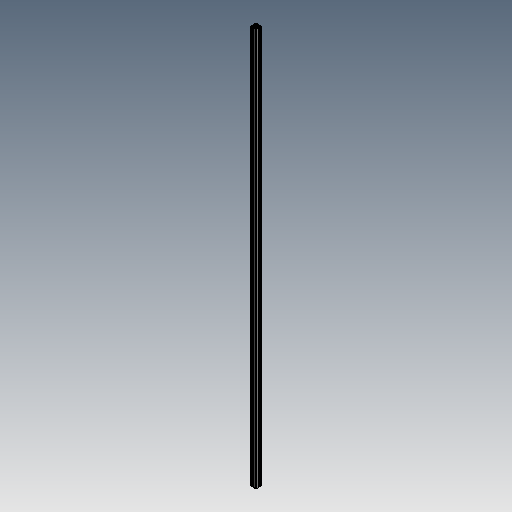
# Autodesk Inventor part: EFS6-3030-2043
Saved by Autodesk Inventor 2020 (Build 240168000, 168)
## iProperties
Part Number: EFS6-3030-2043
Material: 一般
Catalog Web Link: www.cadenas.de
Description: NEFS6-3030, NEFSB6-3030, EFS6-3030, EFSB6-3030, HFS6-3030, HFSB6-3030, CAF6-3030, HFSY6-3030, NFSL6-3030,  HFSL6-3030, HFSLB6-3030, GFS6-3030-HFS6 Series Aluminum Extrusions 30 Square -1 Slot-
Vendor: MISUMI
Document SubType Name: Modeling
Designer: partserver
Manufacturer: MISUMI
Mass: 604.165 g
Surface Area: 6959.94 cm^2
Volume: 604.165 cm^3
Density: 1 g/cm^3
Appearance: PSOLRGB-175-175-175
Category: PARTsolutions
Company: MISUMI
PSOL_IDENT_0: {$CADENAS_DATA\23d-libs\misumi\metric\38_al_extrusions_blackets\6\hfs6_3030.prj},722 {VTYP=3D},{NB=E
PSOL_IDENT_1: FS6-3030-2043},{LINA=EFS6-3030-2043},{NN=NEFS6-3030, NEFSB6-3030, EFS6-3030, EFSB6-3030, HFS6-3030,
PSOL_IDENT_2: HFSB6-3030, CAF6-3030, HFSY6-3030, NFSL6-3030,  HFSL6-3030, HFSLB6-3030, GFS6-3030},{DATE=30.06.2021
PSOL_IDENT_3: 13:36:38},{GEOMDATE=28.10.2014 00:00:00},{VERSION=},{LINEID=150},{WBVAR=L,ALT1,ALT2,ALT3,ALT4,ALT5,
PSOL_IDENT_4: CP5,DL5,DR5,ALT6,ALT9,ALT10,ALT11,DD6SE,DD6,HP6,NHL6,DL6,NHR6,DR6,ALT7,ALT8,NH9,AH,BH,CH,DH,EH,NH10,
PSOL_IDENT_5: AV,BV,CV,DV,EV,NH11,AP,BP,CP,DP,EP,ALT12,ALT13,Z,NH12,XA,XB,XC,XD,XE,NH13,YA,YB,YC,YD,YE,ALT14,HP14,
PSOL_IDENT_6: DL14,DR14,ALT15,HP15,DL15,DR15,ALT16,HP16,DL16,DR16,ALT17,HQ17,JLP,ALT19,ALT20},{WBNUMERIC=L,DD6,NH9
PSOL_IDENT_7: ,AH,BH,CH,DH,EH,NH10,AV,BV,CV,DV,EV,NH11,AP,BP,CP,DP,EP,NH12,XA,XB,XC,XD,XE,NH13,YA,YB,YC,YD,YE,HQ17
PSOL_IDENT_8: ,JLP}  {NB=EFS6-3030-2043},{LINA=EFS6-3030-2043},{KT=DUMMY},{PN=EFS6-3030-2043},{TPS=EFS6-3030},{MAT=
PSOL_IDENT_9: A6N01SS-T5 Aluminum Alloy},{ST=Clear Anodize},{FRMW=30},{FRMH=30},{FRD=6.8},{L=2043.0},{MASS=0.80},{
PSOL_IDENT_10: SA=296},{LX=2.85x10^4},{LY=2.85x10^4},{ALT1=},{M1=0},{IDM1=6.647},{DALT1=4.2},{DPL1=0},{DPR1=0},{ALT
PSOL_IDENT_11: 1PN=},{ALT2=},{ALT2ALG= '','w/o End Tapping (Heli-Coil Insert)','LHP','with LHP (Tapping on the Left
PSOL_IDENT_12: (Heli-Coil Insert))','RHP','with RHP (Tapping on the Right (Heli-Coil Insert))','HPW','with HPW (Ta
PSOL_IDENT_13: pping on Both Ends (Heli-Coil Insert))' },{M2=0},{DP2=0},{ALT2PN=},{ALT3=},{ALT3ALG= '','N/A' },{M3=
PSOL_IDENT_14: 0},{IDM3=4.134},{DP3=0},{ALT3PN=},{ALT4=},{ALT4ALG= '', 'Not applicable' },{ALT4PN=},{ALT5=},{ALT5AL
PSOL_IDENT_15: G= '','w/o 45 Degree Cut','1','with 45 Degree Cut' },{CP5=},{CP5ALG= '','N/A' },{DL5=},{DL5ALG= '','
PSOL_IDENT_16: N/A' },{DR5=},{DR5ALG= '','N/A' },{FRMLALT5=0},{FRMRALT5=0},{ALT5PN=},{ALT6=},{ALT6ALG= '','w/o Fast
PSOL_IDENT_17: ening Location Wrench Access Hole Alterations','1','with Fastening Location Wrench Access Hole Alter
PSOL_IDENT_18: ations' },{ALT9=},{ALT9ALG= '','w/o Location Specified Wrench Access Hole Alteratons (Horizontal)','
PSOL_IDENT_19: 1','with Location Specified Wrench Access Hole Alteratons (Horizontal)' },{ALT10=},{ALT10ALG= '','w/
PSOL_IDENT_20: o Location Specified Wrench Access Hole Alteratons (Vertical)','1','with Location Specified Wrench A
PSOL_IDENT_21: ccess Hole Alteratons (Vertical)' },{ALT11=},{ALT11ALG= '','w/o Location Specified Wrench Access Hol
PSOL_IDENT_22: e Alteratons (Crisscross)','1','with Location Specified Wrench Access Hole Alteratons (Crisscross)'
PSOL_IDENT_23: },{DD6SE=},{DD6SEALG= '','N/A' },{DD6=0},{DD6ALG=0},{HP6=},{HP6ALG= '','N/A' },{NHL6=},{NHL6ALG= '','
PSOL_IDENT_24: N/A' },{DL6=},{DL6ALG= '','N/A' },{NHR6=},{NHR6ALG= '','N/A' },{DR6=},{DR6ALG= '','N/A' },{DD6PN=},{
PSOL_IDENT_25: HL6=0},{HL6D=0},{HR6=0},{HR6D=0},{J6=0},{J6D=0},{K6=0},{K6D=0},{ALT7=},{ALT7ALG= '','N/A' },{ALT8=},
PSOL_IDENT_26: {ALT8ALG= '','N/A' },{ALT678PN=},{NH9=0},{NH9MAX=5},{NH9ALG=[0]},{AH=0.0},{AHMIN=7},{AHMAX=2038},{AH
PSOL_IDENT_27: ALG=[0]},{BH=0.0},{BHMIN=2},{BHMAX=2040},{BHALG=[0]},{CH=0.0},{CHMIN=2},{CHMAX=2042},{CHALG=[0]},{DH=
PSOL_IDENT_28: 0.0},{DHMIN=2},{DHMAX=2044},{DHALG=[0]},{EH=0.0},{EHMIN=2},{EHMAX=2036},{EHALG=[0]},{NH10=0},{NH10MA
PSOL_IDENT_29: X=5},{NH10ALG=[0]},{AV=0.0},{AVMIN=7},{AVMAX=2038},{AVALG=[0]},{BV=0.0},{BVMIN=2},{BVMAX=2040},{BVAL
PSOL_IDENT_30: G=[0]},{CV=0.0},{CVMIN=2},{CVMAX=2042},{CVALG=[0]},{DV=0.0},{DVMIN=2},{DVMAX=2044},{DVALG=[0]},{EV=0
PSOL_IDENT_31: .0},{EVMIN=2},{EVMAX=2036},{EVALG=[0]},{NH11=0},{NH11MAX=5},{NH11ALG=[0]},{AP=0.0},{APMIN=7},{APMAX=
PSOL_IDENT_32: 2038},{APALG=[0]},{BP=0.0},{BPMIN=2},{BPMAX=2040},{BPALG=[0]},{CP=0.0},{CPMIN=2},{CPMAX=2042},{CPALG=
PSOL_IDENT_33: [0]},{DP=0.0},{DPMIN=2},{DPMAX=2044},{DPALG=[0]},{EP=0.0},{EPMIN=2},{EPMAX=2036},{EPALG=[0]},{ALT9PN=
PSOL_IDENT_34: },{ALT10PN=},{ALT11PN=},{ALT91011PN=},{ALT12=},{ALT12ALG= '','w/o Counterbore Hole in Specified Posi
PSOL_IDENT_35: tion (Vertical)','1','with Counterbore Hole in Specified Position (Vertical)' },{ALT13=},{ALT13ALG= ''
PSOL_IDENT_36: ,'w/o Counterbore Hole in Specified Position (Horizontal)','1','with Counterbore Hole in Specified P
PSOL_IDENT_37: osition (Horizontal)' },{Z=},{ZALG= '','N/A' },{DD12=0.0},{DD112=0.0},{NH12=0},{NH12MAX=5},{NH12ALG=
PSOL_IDENT_38: [0]},{XA=0.0},{XAMIN=7},{XAMAX=2038},{XAALG=[0]},{XB=0.0},{XBMIN=2},{XBMAX=2040},{XBALG=[0]},{XC=0.0
PSOL_IDENT_39: },{XCMIN=2},{XCMAX=2042},{XCALG=[0]},{XD=0.0},{XDMIN=2},{XDMAX=2044},{XDALG=[0]},{XE=0.0},{XEMIN=2},
PSOL_IDENT_40: {XEMAX=2036},{XEALG=[0]},{NH13=0},{NH13MAX=5},{NH13ALG=[0]},{YA=0.0},{YAMIN=7},{YAMAX=2038},{YAALG=[
PSOL_IDENT_41: 0]},{YB=0.0},{YBMIN=2},{YBMAX=2040},{YBALG=[0]},{YC=0.0},{YCMIN=2},{YCMAX=2042},{YCALG=[0]},{YD=0.0}
PSOL_IDENT_42: ,{YDMIN=2},{YDMAX=2044},{YDALG=[0]},{YE=0.0},{YEMIN=2},{YEMAX=2036},{YEALG=[0]},{ALT12PN=},{ALT13PN=
PSOL_IDENT_43: },{ALT1213PN=},{ALT14=},{ALT14ALG= '','w/o D Type Hole Alteration','1','with D Type Hole Alteration'
PSOL_IDENT_44: },{HP14=},{HP14ALG= '','N/A' },{DL14=},{DL14ALG= '','N/A' },{DR14=},{DR14ALG= '','N/A' },{H14=0},{D
PSOL_IDENT_45: 14=0.0},{ALT14PN=},{ALT15=},{ALT15ALG= '','w/o S Type Hole Alteration','1','with S Type Hole Alterat
PSOL_IDENT_46: ion' },{HP15=},{HP15ALG= '','N/A' },{DL15=},{DL15ALG= '','N/A' },{DR15=},{DR15ALG= '','N/A' },{H15=0
PSOL_IDENT_47: },{D115=0.0},{D215=0.0},{ALT15PN=},{ALT16=},{ALT16ALG= '','w/o M Type Hole Alteration','1','with M T
PSOL_IDENT_48: ype Hole Alteration' },{HP16=},{HP16ALG= '','N/A' },{DL16=},{DL16ALG= '','N/A' },{DR16=},{DR16ALG= ''
PSOL_IDENT_49: ,'N/A' },{H116=0},{D16=0.0},{ALT16PN=},{ALT17=},{ALT17ALG= '','w/o L Type Hole Alteration (Top)','1'
PSOL_IDENT_50: ,'with L Type Hole Alteration (Top)' },{HQ17=0},{HQ17ALG=0},{JLP=0},{JLPMIN=4.9},{JLPMAX=0},{JLPALG=
PSOL_IDENT_51: [0]},{L17=0},{D17=0.0},{ALT17PN=},{ALT19=},{ALT19ALG= '','N/A' },{M19=0},{DP19=0},{ALT19PN=},{ALT20=
PSOL_IDENT_52: },{ALT20PN=},{ERRORALT01=OK},{ERRORALT02=OK},{ERRORALT03=OK},{ERRORALT05=OK},{ERRORALT06091=OK},{ERR
PSOL_IDENT_53: ORALT06092=OK},{ERRORALT06093=OK},{ERRORALT06094=OK},{ERRORALT06101=OK},{ERRORALT06102=OK},{ERRORALT
PSOL_IDENT_54: 06103=OK},{ERRORALT06104=OK},{ERRORALT06111=OK},{ERRORALT06112=OK},{ERRORALT06113=OK},{ERRORALT06114=
PSOL_IDENT_55: OK},{ERRORALT06121=OK},{ERRORALT06122=OK},{ERRORALT06123=OK},{ERRORALT06124=OK},{ERRORALT06131=OK},{
PSOL_IDENT_56: ERRORALT06132=OK},{ERRORALT06133=OK},{ERRORALT06134=OK},{ERRORALT0614=OK},{ERRORALT0615=OK},{ERRORAL
PSOL_IDENT_57: T0616=OK},{ERRORALT06171=OK},{ERRORALT06172=OK},{ERRORALT06173=OK},{ERRORALT0619=OK},{ERRORALT0911=O
PSOL_IDENT_58: K},{ERRORALT0913=OK},{ERRORALT0914=OK},{ERRORALT0915=OK},{ERRORALT0916=OK},{ERRORALT0917=OK},{ERRORA
PSOL_IDENT_59: LT0919=OK},{ERRORALT1011=OK},{ERRORALT1012=OK},{ERRORALT1014=OK},{ERRORALT1015=OK},{ERRORALT1016=OK}
PSOL_IDENT_60: ,{ERRORALT1017=OK},{ERRORALT1019=OK},{ERRORALT1112=OK},{ERRORALT1113=OK},{ERRORALT1114=OK},{ERRORALT
PSOL_IDENT_61: 1115=OK},{ERRORALT1116=OK},{ERRORALT1117=OK},{ERRORALT1119=OK},{ERRORALT1214=OK},{ERRORALT1215=OK},{
PSOL_IDENT_62: ERRORALT1216=OK},{ERRORALT1217=OK},{ERRORALT1219=OK},{ERRORALT1314=OK},{ERRORALT1315=OK},{ERRORALT13
PSOL_IDENT_63: 16=OK},{ERRORALT1317=OK},{ERRORALT1319=OK},{ERRORALT1415=OK},{ERRORALT1416=OK},{ERRORALT1417=OK},{ER
PSOL_IDENT_64: RORALT1419=OK},{ERRORALT1516=OK},{ERRORALT1517=OK},{ERRORALT1519=OK},{ERRORALT1617=OK},{ERRORALT1619=
PSOL_IDENT_65: OK},{ERRORALT1719=OK},{ERRORPN=}
NB: EFS6-3030-2043
NN: NEFS6-3030, NEFSB6-3030, EFS6-3030, EFSB6-3030, HFS6-3030, HFSB6-3030, CAF6-3030, HFSY6-3030, NFSL6-3030,  HFSL6-3030, HFSLB6-3030, GFS6-3030
NT: HFS6 Series Aluminum Extrusions 30 Square -1 Slot-
NBSYN: $PN.
LINA: EFS6-3030-2043
CATALOG: Misumi
PN: EFS6-3030-2043
TPS: EFS6-3030
MAT: A6N01SS-T5 Aluminum Alloy
ST: Clear Anodize
L: 2043
MASS: 0.80
SA: 296
LX: 2.85x10^4
LY: 2.85x10^4
ALT1: w/o End Tapping
M1: 0
DPL1: 0
DPR1: 0
ALT2: w/o End Tapping (Heli-Coil Insert)
M2: 0
DP2: 0
ALT3: N/A
M3: 0
DP3: 0
ALT4: Not applicable
ALT5: w/o 45 Degree Cut
CP5: N/A
DL5: N/A
DR5: N/A
ALT6: w/o Fastening Location Wrench Access Hole Alterations
ALT9: w/o Location Specified Wrench Access Hole Alteratons (Horizontal)
ALT10: w/o Location Specified Wrench Access Hole Alteratons (Vertical)
ALT11: w/o Location Specified Wrench Access Hole Alteratons (Crisscross)
DD6SE: N/A
DD6: 0
HP6: N/A
NHL6: N/A
DL6: N/A
NHR6: N/A
DR6: N/A
HL6D: 0
HR6D: 0
J6D: 0
K6D: 0
ALT7: N/A
ALT8: N/A
NH9: 0
AH: 0
BH: 0
CH: 0
DH: 0
EH: 0
NH10: 0
AV: 0
BV: 0
CV: 0
DV: 0
EV: 0
NH11: 0
AP: 0
BP: 0
CP: 0
DP: 0
EP: 0
ALT12: w/o Counterbore Hole in Specified Position (Vertical)
ALT13: w/o Counterbore Hole in Specified Position (Horizontal)
Z: N/A
DD12: 0
DD112: 0
NH12: 0
XA: 0
XB: 0
XC: 0
XD: 0
XE: 0
NH13: 0
YA: 0
YB: 0
YC: 0
YD: 0
YE: 0
ALT14: w/o D Type Hole Alteration
HP14: N/A
DL14: N/A
DR14: N/A
H14: 0
D14: 0
ALT15: w/o S Type Hole Alteration
HP15: N/A
DL15: N/A
DR15: N/A
H15: 0
D115: 0
D215: 0
ALT16: w/o M Type Hole Alteration
HP16: N/A
DL16: N/A
DR16: N/A
H116: 0
D16: 0
ALT17: w/o L Type Hole Alteration (Top)
HQ17: 0
JLP: 0
D17: 0
ALT19: N/A
M19: 0
DP19: 0
ALT20: w/o CW (End Face C Chamfering)
SUPPLIER: MISUMI
ARTICLENO: EFS6-3030-2043
BOMINFO: EFS6-3030-2043
CREATOR: CADENAS GmbH
Title: EFS6-3030-2043
Author: Cadenas PARTsolutions
Comments: HFS6 Series Aluminum Extrusions 30 Square -1 Slot-
Autodesk Inventor part; units mm, degrees
sketch "Sketch_2" plane through (0, 0, 0) normal (0, 0, 1) x (1, 0, 0)
  line L0 (-15, -4) -> (-15, -13)
  arc A0 (-15, -13) -> (-13, -15) centre (-13, -13) ccw
  line L1 (-13, -15) -> (-4, -15)
  line L2 (-4, -15) -> (-4, -13)
  line L3 (-4, -13) -> (-8.25, -13)
  line L4 (-8.25, -13) -> (-8.25, -9.6642)
  line L5 (-8.25, -9.6642) -> (-4.5858, -6)
  line L6 (-4.5858, -6) -> (-2.7434, -6)
  line L7 (-2.7434, -6) -> (-1.2, -5.7)
  line L8 (-1.2, -5.7) -> (-0.75, -5.9598)
  arc A1 (-0.75, -5.9598) -> (-0.45, -5.9598) centre (-0.6, -5.7) ccw
  line L9 (-0.45, -5.9598) -> (0, -5.7)
  line L10 (0, -5.7) -> (0.45, -5.9598)
  arc A2 (0.45, -5.9598) -> (0.75, -5.9598) centre (0.6, -5.7) ccw
  line L11 (0.75, -5.9598) -> (1.2, -5.7)
  line L12 (1.2, -5.7) -> (2.7434, -6)
  line L13 (2.7434, -6) -> (4.5858, -6)
  line L14 (4.5858, -6) -> (8.25, -9.6642)
  line L15 (8.25, -9.6642) -> (8.25, -13)
  line L16 (8.25, -13) -> (4, -13)
  line L17 (4, -13) -> (4, -15)
  line L18 (4, -15) -> (13, -15)
  arc A3 (13, -15) -> (15, -13) centre (13, -13) ccw
  line L19 (15, -13) -> (15, -4)
  line L20 (15, -4) -> (13, -4)
  line L21 (13, -4) -> (13, -8.25)
  line L22 (13, -8.25) -> (9.6642, -8.25)
  line L23 (9.6642, -8.25) -> (6, -4.5858)
  line L24 (6, -4.5858) -> (6, -2.7434)
  line L25 (6, -2.7434) -> (5.7, -1.2)
  line L26 (5.7, -1.2) -> (5.9598, -0.75)
  arc A4 (5.9598, -0.75) -> (5.9598, -0.45) centre (5.7, -0.6) ccw
  line L27 (5.9598, -0.45) -> (5.7, 0)
  line L28 (5.7, 0) -> (5.9598, 0.45)
  arc A5 (5.9598, 0.45) -> (5.9598, 0.75) centre (5.7, 0.6) ccw
  line L29 (5.9598, 0.75) -> (5.7, 1.2)
  line L30 (5.7, 1.2) -> (6, 2.7434)
  line L31 (6, 2.7434) -> (6, 4.5858)
  line L32 (6, 4.5858) -> (9.6642, 8.25)
  line L33 (9.6642, 8.25) -> (13, 8.25)
  line L34 (13, 8.25) -> (13, 4)
  line L35 (13, 4) -> (15, 4)
  line L36 (15, 4) -> (15, 13)
  arc A6 (15, 13) -> (13, 15) centre (13, 13) ccw
  line L37 (13, 15) -> (4, 15)
  line L38 (4, 15) -> (4, 13)
  line L39 (4, 13) -> (8.25, 13)
  line L40 (8.25, 13) -> (8.25, 9.6642)
  line L41 (8.25, 9.6642) -> (4.5858, 6)
  line L42 (4.5858, 6) -> (2.7434, 6)
  line L43 (2.7434, 6) -> (1.2, 5.7)
  line L44 (1.2, 5.7) -> (0.75, 5.9598)
  arc A7 (0.75, 5.9598) -> (0.45, 5.9598) centre (0.6, 5.7) ccw
  line L45 (0.45, 5.9598) -> (0, 5.7)
  line L46 (0, 5.7) -> (-0.45, 5.9598)
  arc A8 (-0.45, 5.9598) -> (-0.75, 5.9598) centre (-0.6, 5.7) ccw
  line L47 (-0.75, 5.9598) -> (-1.2, 5.7)
  line L48 (-1.2, 5.7) -> (-2.7434, 6)
  line L49 (-2.7434, 6) -> (-4.5858, 6)
  line L50 (-4.5858, 6) -> (-8.25, 9.6642)
  line L51 (-8.25, 9.6642) -> (-8.25, 13)
  line L52 (-8.25, 13) -> (-4, 13)
  line L53 (-4, 13) -> (-4, 15)
  line L54 (-4, 15) -> (-13, 15)
  arc A9 (-13, 15) -> (-15, 13) centre (-13, 13) ccw
  line L55 (-15, 13) -> (-15, 4)
  line L56 (-15, 4) -> (-13, 4)
  line L57 (-13, 4) -> (-13, 8.25)
  line L58 (-13, 8.25) -> (-9.6642, 8.25)
  line L59 (-9.6642, 8.25) -> (-6, 4.5858)
  line L60 (-6, 4.5858) -> (-6, 2.7434)
  line L61 (-6, 2.7434) -> (-5.7, 1.2)
  line L62 (-5.7, 1.2) -> (-5.9598, 0.75)
  arc A10 (-5.9598, 0.75) -> (-5.9598, 0.45) centre (-5.7, 0.6) ccw
  line L63 (-5.9598, 0.45) -> (-5.7, 0)
  line L64 (-5.7, 0) -> (-5.9598, -0.45)
  arc A11 (-5.9598, -0.45) -> (-5.9598, -0.75) centre (-5.7, -0.6) ccw
  line L65 (-5.9598, -0.75) -> (-5.7, -1.2)
  line L66 (-5.7, -1.2) -> (-6, -2.7434)
  line L67 (-6, -2.7434) -> (-6, -4.5858)
  line L68 (-6, -4.5858) -> (-9.6642, -8.25)
  line L69 (-9.6642, -8.25) -> (-13, -8.25)
  line L70 (-13, -8.25) -> (-13, -4)
  line L71 (-13, -4) -> (-15, -4)
  arc A12 (9.5391, 11.3389) -> (11.3389, 9.5391) centre (10.8515, 10.8515) ccw
  line L72 (11.3389, 9.5391) -> (12.3615, 9.9189)
  arc A13 (12.3615, 9.9189) -> (9.9189, 12.3615) centre (11.7, 11.7) ccw
  line L73 (9.9189, 12.3615) -> (9.5391, 11.3389)
  arc A14 (11.3389, -9.5391) -> (9.5391, -11.3389) centre (10.8515, -10.8515) ccw
  line L74 (9.5391, -11.3389) -> (9.9189, -12.3615)
  arc A15 (9.9189, -12.3615) -> (12.3615, -9.9189) centre (11.7, -11.7) ccw
  line L75 (12.3615, -9.9189) -> (11.3389, -9.5391)
  arc A16 (-9.9189, 12.3615) -> (-12.3615, 9.9189) centre (-11.7, 11.7) ccw
  line L76 (-12.3615, 9.9189) -> (-11.3389, 9.5391)
  arc A17 (-11.3389, 9.5391) -> (-9.5391, 11.3389) centre (-10.8515, 10.8515) ccw
  line L77 (-9.5391, 11.3389) -> (-9.9189, 12.3615)
  arc A18 (-12.3615, -9.9189) -> (-9.9189, -12.3615) centre (-11.7, -11.7) ccw
  line L78 (-9.9189, -12.3615) -> (-9.5391, -11.3389)
  arc A19 (-9.5391, -11.3389) -> (-11.3389, -9.5391) centre (-10.8515, -10.8515) ccw
  line L79 (-11.3389, -9.5391) -> (-12.3615, -9.9189)
  constraints: 160 end point, 40 point on circle, 20 centre point
extrude "Extrusion1" add sketch "Sketch_2" against normal blind 2043
sketch "Sketch_91" plane through (0, 0, 0) normal (0, 0, 1) x (1, 0, 0)
  arc A0 (-4.8, 2.6444) -> (-4.7945, 2.5872) centre (-4.5, 2.6444) ccw
  line L0 (-4.7945, 2.5872) -> (-4.6303, 1.7428)
  arc A1 (-4.6303, 1.7428) -> (-4.3359, 1.5) centre (-4.3359, 1.8) ccw
  line L1 (-4.3359, 1.5) -> (-3.5, 1.5)
  arc A2 (-3.2162, 1.1027) -> (-3.5, 1.5) centre (-3.5, 1.2) ccw
  arc A3 (-3.2162, 1.1027) -> (-3.2162, -1.1027) centre (0, 0) ccw
  arc A4 (-3.5, -1.5) -> (-3.2162, -1.1027) centre (-3.5, -1.2) ccw
  line L2 (-3.5, -1.5) -> (-4.3359, -1.5)
  arc A5 (-4.3359, -1.5) -> (-4.6303, -1.7428) centre (-4.3359, -1.8) ccw
  line L3 (-4.6303, -1.7428) -> (-4.7945, -2.5872)
  arc A6 (-4.7945, -2.5872) -> (-4.8, -2.6444) centre (-4.5, -2.6444) ccw
  line L4 (-4.8, -2.6444) -> (-4.8, -4.5)
  arc A7 (-4.8, -4.5) -> (-4.5, -4.8) centre (-4.5, -4.5) ccw
  line L5 (-4.5, -4.8) -> (-2.6444, -4.8)
  arc A8 (-2.6444, -4.8) -> (-2.5872, -4.7945) centre (-2.6444, -4.5) ccw
  line L6 (-2.5872, -4.7945) -> (-1.7428, -4.6303)
  arc A9 (-1.7428, -4.6303) -> (-1.5, -4.3359) centre (-1.8, -4.3359) ccw
  line L7 (-1.5, -4.3359) -> (-1.5, -3.5)
  arc A10 (-1.1027, -3.2162) -> (-1.5, -3.5) centre (-1.2, -3.5) ccw
  arc A11 (-1.1027, -3.2162) -> (1.1027, -3.2162) centre (0, 0) ccw
  arc A12 (1.5, -3.5) -> (1.1027, -3.2162) centre (1.2, -3.5) ccw
  line L8 (1.5, -3.5) -> (1.5, -4.3359)
  arc A13 (1.5, -4.3359) -> (1.7428, -4.6303) centre (1.8, -4.3359) ccw
  line L9 (1.7428, -4.6303) -> (2.5872, -4.7945)
  arc A14 (2.5872, -4.7945) -> (2.6444, -4.8) centre (2.6444, -4.5) ccw
  line L10 (2.6444, -4.8) -> (4.5, -4.8)
  arc A15 (4.5, -4.8) -> (4.8, -4.5) centre (4.5, -4.5) ccw
  line L11 (4.8, -4.5) -> (4.8, -2.6444)
  arc A16 (4.8, -2.6444) -> (4.7945, -2.5872) centre (4.5, -2.6444) ccw
  line L12 (4.7945, -2.5872) -> (4.6303, -1.7428)
  arc A17 (4.6303, -1.7428) -> (4.3359, -1.5) centre (4.3359, -1.8) ccw
  line L13 (4.3359, -1.5) -> (3.5, -1.5)
  arc A18 (3.2162, -1.1027) -> (3.5, -1.5) centre (3.5, -1.2) ccw
  arc A19 (3.2162, -1.1027) -> (3.2162, 1.1027) centre (0, 0) ccw
  arc A20 (3.5, 1.5) -> (3.2162, 1.1027) centre (3.5, 1.2) ccw
  line L14 (3.5, 1.5) -> (4.3359, 1.5)
  arc A21 (4.3359, 1.5) -> (4.6303, 1.7428) centre (4.3359, 1.8) ccw
  line L15 (4.6303, 1.7428) -> (4.7945, 2.5872)
  arc A22 (4.7945, 2.5872) -> (4.8, 2.6444) centre (4.5, 2.6444) ccw
  line L16 (4.8, 2.6444) -> (4.8, 4.5)
  arc A23 (4.8, 4.5) -> (4.5, 4.8) centre (4.5, 4.5) ccw
  line L17 (4.5, 4.8) -> (2.6444, 4.8)
  arc A24 (2.6444, 4.8) -> (2.5872, 4.7945) centre (2.6444, 4.5) ccw
  line L18 (2.5872, 4.7945) -> (1.7428, 4.6303)
  arc A25 (1.7428, 4.6303) -> (1.5, 4.3359) centre (1.8, 4.3359) ccw
  line L19 (1.5, 4.3359) -> (1.5, 3.5)
  arc A26 (1.1027, 3.2162) -> (1.5, 3.5) centre (1.2, 3.5) ccw
  arc A27 (1.1027, 3.2162) -> (-1.1027, 3.2162) centre (0, 0) ccw
  arc A28 (-1.5, 3.5) -> (-1.1027, 3.2162) centre (-1.2, 3.5) ccw
  line L20 (-1.5, 3.5) -> (-1.5, 4.3359)
  arc A29 (-1.5, 4.3359) -> (-1.7428, 4.6303) centre (-1.8, 4.3359) ccw
  line L21 (-1.7428, 4.6303) -> (-2.5872, 4.7945)
  arc A30 (-2.5872, 4.7945) -> (-2.6444, 4.8) centre (-2.6444, 4.5) ccw
  line L22 (-2.6444, 4.8) -> (-4.5, 4.8)
  arc A31 (-4.5, 4.8) -> (-4.8, 4.5) centre (-4.5, 4.5) ccw
  line L23 (-4.8, 4.5) -> (-4.8, 2.6444)
  constraints: 64 point on circle, 48 end point, 32 centre point
extrude "Extrusion2" cut sketch "Sketch_91" against normal blind 2043
ref_plane "C1_XY" through (0, 0, 0) normal (0, 0, 1) x (1, 0, 0)
ref_plane "C1_YZ" through (0, 0, 0) normal (1, 0, 0) x (0, 1, 0)
ref_plane "C1_ZX" through (0, 0, 0) normal (0, 1, 0) x (0, 0, 1)
ref_plane "to_frame_cap1_XY" through (0, 0, 0) normal (0, 0, 1) x (1, 0, 0)
ref_plane "to_frame_cap1_YZ" through (0, 0, 0) normal (1, 0, 0) x (0, 1, 0)
ref_plane "to_frame_cap1_ZX" through (0, 0, 0) normal (0, 1, 0) x (0, 0, 1)
ref_plane "to_frame_cap2_XY" through (0, 0, -2043) normal (0, 0, -1) x (1, 0, 0)
ref_plane "to_frame_cap2_YZ" through (0, 0, -2043) normal (1, 0, 0) x (0, -1, 0)
ref_plane "to_frame_cap2_ZX" through (0, 0, -2043) normal (0, -1, 0) x (0, 0, -1)
body "Solid1"
